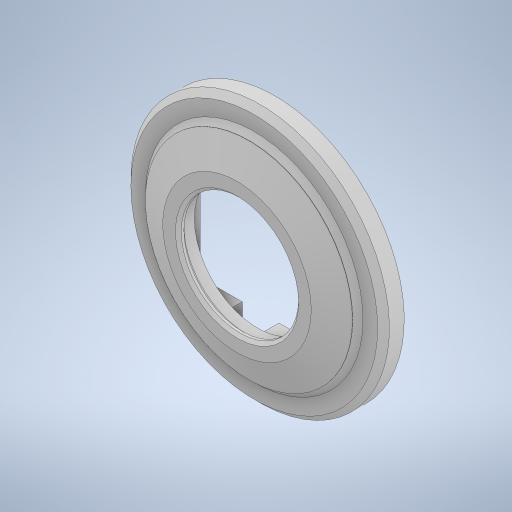
# Autodesk Inventor part: controls_knob_cover
Saved by Autodesk Inventor 2023 (Build 270158000, 158)
## iProperties
Created: 2023-12-03
Part Number: controls_knob_cover
Material: Generic
Document SubType Name: Modeling
Designer: aaron
Density: 1 g/cm^3
Appearance: Default
Author: aaron
Autodesk Inventor part; units mm, degrees
ref_plane "YZ Plane" through (0, 0, 0) normal (1, 0, 0) x (0, 1, 0)
ref_plane "XZ Plane" through (0, 0, 0) normal (0, 1, 0) x (-1, 0, 0)
ref_plane "XY Plane" through (0, 0, 0) normal (0, 0, 1) x (1, 0, 0)
sketch "Sketch1" plane through (0, 0, 0) normal (0, 0, 1) x (1, 0, 0)
  circle A0 centre (0, 0) radius 33.25
  circle A1 centre (0, 0) radius 26.475
  circle A2 centre (0, 0) radius 35.25
  dimension "d0" = 66.5
  dimension "d1" = 52.95
  dimension "d2" = 2
  constraints: 3 centre point, 2 coincident
  measures "d0" diameter of A0
  measures "d1" diameter of A1
  measures "d2" radial gap between concentric circles of A0 A2
extrude "Extrusion1" add sketch "Sketch1" along normal blind 10.35
sketch "Sketch2" plane through (0, 0, 10.35) normal (0, 0, 1) x (1, 0, 0)
  circle A0 centre (0, 0) radius 35.25 projected
extrude "Extrusion2" add sketch "Sketch2" against normal blind 0.5
sketch "Sketch3" plane through (0, 0, 10.35) normal (0, 0, 1) x (1, 0, 0)
  circle A0 centre (0, 0) radius 16
  dimension "d7" = 32
  constraints: 1 centre point, 1 coincident
  measures "d7" diameter of A0
extrude "Extrusion3" cut sketch "Sketch3" against normal blind 2.5
sketch "Sketch4" plane through (0, 0, 7.85) normal (0, 0, 1) x (1, 0, 0)
  circle A0 centre (0, 0) radius 17.25
  dimension "d10" = 34.5
  constraints: 1 centre point, 1 coincident
  measures "d10" diameter of A0
extrude "Extrusion4" cut sketch "Sketch4" against normal blind 3.1
sketch "Sketch5" plane through (0, 0, 4.75) normal (0, 0, 1) x (1, 0, 0)
  line L0 (-20.4, 17.85) -> (20.4, 17.85)
  line L1 (20.4, 17.85) -> (20.4, -17.85)
  line L2 (20.4, -17.85) -> (-20.4, -17.85)
  line L3 (-20.4, -17.85) -> (-20.4, 17.85)
  point P0 (0, 0)
  dimension "d13" = 40.8
  dimension "d14" = 35.7
  dimension "d15" = 17.85
  dimension "d16" = 20.4
  constraints: 8 end point, 2 parallel, 1 horizontal, 1 perpendicular
  measures "d13" distance of L1.end L2.end
  measures "d14" distance of L0.end L1.end
  measures "d15" distance from line of L2 point (0, 0)
  measures "d16" distance from line of L1 point (0, 0)
extrude "Extrusion5" cut sketch "Sketch5" against normal through all
chamfer "Chamfer1" distance 0.8 angle 45 1 edges at (-16, 0, 10.35)
sketch "Sketch6" plane through (0, 0, 9.85) normal (0, 0, -1) x (-1, 0, 0)
  circle A0 centre (0, 0) radius 33.25 projected
  circle A1 centre (0, 0) radius 26.475 projected
extrude "Extrusion6" add sketch "Sketch6" along normal up to surface (5.1 mm away)
chamfer "Chamfer4" distance 1 angle 45 1 edges at (-16, 0, 7.85)
sketch "Sketch7" plane through (0, 0, 0) normal (0, 0, -1) x (-1, 0, 0)
  line L0 (8.9, -41.2726) -> (-1.1, -41.2726)
  line L1 (-1.1, -41.2726) -> (-1.1, 4.8372)
  line L2 (-1.1, 4.8372) -> (8.9, 4.8372)
  line L3 (8.9, 4.8372) -> (8.9, -41.2726)
  line L4 (19.5526, -17.85) -> (-19.5526, -17.85) projected
  line L5 (-20.4, -16.875) -> (-20.4, 16.875) projected
  line L6 (20.4, 16.875) -> (20.4, -16.875) projected
  point P0 (0, 0)
  point P1 (3.9, -41.2726)
  dimension "d36" = 10
  dimension "d40" = 21.5
  constraints: 8 end point, 2 parallel, 1 horizontal, 1 midpoint, 1 perpendicular
  measures "d36" distance of L0.start L0.end
  measures "d40" distance between parallel lines of L6 L1
extrude "Extrusion7" cut sketch "Sketch7" against normal up to surface (4.75 mm away)
sketch "Sketch8" plane through (0, 0, 10.35) normal (0, 0, 1) x (1, 0, 0)
  circle A0 centre (0, 0) radius 35.25 projected
  circle A1 centre (0, 0) radius 28.25
  dimension "d41" = 7
  constraints: 1 centre point
  measures "d41" radial gap between concentric circles of A0 A1
extrude "Extrusion8" cut sketch "Sketch8" against normal blind 4.7
chamfer "Chamfer5" distance 8 angle 22 1 edges at (-28.25, 0, 10.35) measured on face at (23.997, -3.5937, 10.35)
chamfer "Chamfer6" distance 1.6 angle 45 1 edges at (-35.25, 0, 5.65)
chamfer "Chamfer7" distance 1.4 angle 45 1 edges at (-28.25, 0, 5.65)
equation "\"d15\" = 0.5 * d14"
equation "\"d16\" = 0.5 * d13"
body "Solid1"
